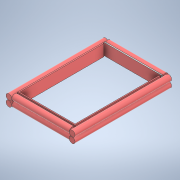
# Autodesk Inventor part: bumper
Saved by Autodesk Inventor 2022 (Build 260153000, 153)
## iProperties
Created: 2023-01-11
Part Number: bumper
Material: Generic
Document SubType Name: Modeling
Designer: s135320
Density: 1 g/cm^3
Appearance: Default
Author: s135320
Autodesk Inventor part; units mm, degrees
ref_plane "YZ Plane" through (0, 0, 0) normal (1, 0, 0) x (0, 1, 0)
ref_plane "XZ Plane" through (0, 0, 0) normal (0, 1, 0) x (-1, 0, 0)
ref_plane "XY Plane" through (0, 0, 0) normal (0, 0, 1) x (1, 0, 0)
sketch "Sketch2" plane through (0, 0, 0) normal (0, 0, 1) x (1, 0, 0)
  line L0 (0, 0) -> (-12.7, 0)
  line L1 (-12.7, 0) -> (-12.7, 127)
  line L2 (-12.7, 127) -> (0, 127)
  line L3 (0, 127) -> (0, 0)
  line L4 (0, 63.5) -> (0, 0)
  line L5 (0, 63.5) -> (0, 127)
  line L6 (0, 95.25) -> (31.75, 95.25)
  line L7 (0, 31.75) -> (31.75, 31.75)
  circle A0 centre (31.75, 31.75) radius 31.75
  circle A1 centre (31.75, 95.25) radius 31.75
  line L8 (-317.5, 0) -> (-317.5, 211.5166)
  line L9 (-635, 0) -> (-622.3, 0)
  line L10 (-622.3, 0) -> (-622.3, 127)
  line L11 (-622.3, 127) -> (-635, 127)
  line L12 (-635, 127) -> (-635, 0)
  circle A2 centre (-666.75, 31.75) radius 31.75
  circle A3 centre (-666.75, 95.25) radius 31.75
  point P0 (31.75, 63.5)
  point P1 (-666.75, 63.5)
  point P2 (-635, 31.75)
  point P3 (-635, 95.25)
  dimension "d0" = 12.7
  dimension "d1" = 127
  dimension "d2" = 31.75
  dimension "d13" = 304.8
  constraints: 26 end point, 6 symmetric about line, 3 horizontal, 3 midpoint, 2 centre point, 2 coincident, 2 collinear, 2 parallel, 1 perpendicular, 1 vertical, 8 other
  measures "d0" distance of L1.end L2.end
  measures "d1" distance of L0.end L1.end
  measures "d2" distance of L6.start L6.end
  measures "d13" distance between parallel lines of L1 L8
extrude "Extrusion1" add sketch "Sketch2" along normal blind 939.8 contours L0 L1 L2 L3 | A0 | A1 | L12 L11 L10 L9 | A2 | A3
extrude "Extrusion2" add sketch "Sketch2" against normal blind 63.5 contours A0 | A1 | A2 | A3
sketch "Sketch4" plane through (0, 0, 939.8) normal (0, 0, 1) x (1, 0, 0)
  circle A0 centre (31.75, 31.75) radius 31.75 projected
  circle A1 centre (31.75, 31.75) radius 31.75
  circle A2 centre (31.75, 95.25) radius 31.75 projected
  circle A3 centre (31.75, 95.25) radius 31.75
  line L0 (-317.5, 0) -> (-317.5, 256.9673)
  line L1 (-12.7, 127) -> (-12.7, 0) projected
  circle A4 centre (-666.75, 31.75) radius 31.75
  circle A5 centre (-666.75, 95.25) radius 31.75
  point P0 (0, 0)
  point P1 (31.75, 63.5)
  point P2 (-666.75, 63.5)
  dimension "d14" = 304.8
  constraints: 4 centre point, 2 coincident, 2 end point, 2 symmetric about line, 2 vertical alignment, 1 vertical, 2 other
  measures "d14" distance between parallel lines of L1 L0
extrude "Extrusion3" add sketch "Sketch4" along normal blind 63.5
sketch "Sketch5" plane through (-12.7, 0, 0) normal (-1, 0, 0) x (0, 0, 1)
  point P0 (0, 0)
sketch "Sketch6" plane through (0, 95.25, 0) normal (1, 0, 0) x (0, 0, -1)
  line L0 (-939.8, 31.75) -> (-939.8, -95.25) projected
  line L1 (-939.8, 31.75) -> (-927.1, 31.75)
  line L2 (-927.1, 31.75) -> (-927.1, -95.25)
  line L3 (-927.1, -95.25) -> (-939.8, -95.25)
  line L4 (-939.8, -95.25) -> (-939.8, 31.75)
  line L5 (0, 0) -> (-939.8, 0) projected
  line L6 (-939.8, 0) -> (-971.55, 0)
  line L7 (0, -63.5) -> (-939.8, -63.5) projected
  line L8 (-939.8, -63.5) -> (-971.55, -63.5)
  circle A0 centre (-971.55, 0) radius 31.75
  circle A1 centre (-971.55, -63.5) radius 31.75
  line L9 (-457.2, 0) -> (-457.2, 166.6029)
  line L10 (0, 31.75) -> (0, -95.25) projected
  line L11 (25.4, 31.75) -> (25.4, -95.25)
  line L12 (25.4, 31.75) -> (12.7, 31.75)
  line L13 (12.7, 31.75) -> (12.7, -95.25)
  line L14 (12.7, -95.25) -> (25.4, -95.25)
  circle A2 centre (57.15, 0) radius 31.75
  circle A3 centre (57.15, -63.5) radius 31.75
  point P0 (-971.55, -31.75)
  point P1 (57.15, -31.75)
  dimension "d9" = 12.7
  dimension "d10" = 31.75
  dimension "d15" = 457.2
  dimension "d16" = 12.7
  dimension "d17" = 31.75
  dimension "d18" = 31.75
  constraints: 22 end point, 7 symmetric about line, 3 horizontal, 2 centre point, 2 coincident, 2 parallel, 1 perpendicular, 1 vertical, 8 other
  measures "d9" distance of L2.end L3.end
  measures "d10" distance of L5.end L6.end
  measures "d15" distance between parallel lines of L10 L9
  measures "d16" distance of L12.start L13.start
  measures "d17" distance from line of L11 A2.centre
  measures "d18" distance from line of L11 A3.centre
extrude "Extrusion4" add sketch "Sketch6" against normal blind 635 contours L1 L2 L5 L0 | L5 L2 L7 L0 | A0 | L7 L2 L3 L0 | A1 | L11 L14 L13 L12 | A2 | A3
body "Solid1"
